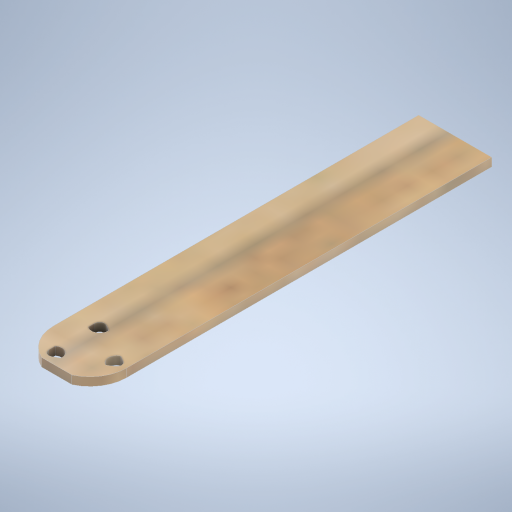
# Autodesk Inventor part: dish_upper
Saved by Autodesk Inventor 2024.1 (Build 281209000, 209)
## iProperties
Created: 2025-09-27
Part Number: dish_upper
Material: 木材 (カエデ材)
Document SubType Name: Modeling
Designer: hibik
Density: 0.67 g/cm^3
Appearance: ナチュラル カエデ材 - 光沢 濃い着色
Author: hibik
Autodesk Inventor part; units mm, degrees
ref_plane "YZ Plane" through (0, 0, 0) normal (1, 0, 0) x (0, 1, 0)
ref_plane "XZ Plane" through (0, 0, 0) normal (0, 1, 0) x (-1, 0, 0)
ref_plane "XY Plane" through (0, 0, 0) normal (0, 0, 1) x (1, 0, 0)
sketch "スケッチ1" plane through (0, 0, 0) normal (0, 1, 0) x (-1, 0, 0)
  circle A0 centre (0, 0) radius 11
  line L0 (11, 10) -> (-11, 10)
  line L1 (-11, 10) -> (-11, -10)
  line L2 (-11, -10) -> (11, -10)
  line L3 (11, -10) -> (11, 10)
  line L4 (11, -10) -> (-11, -10)
  line L5 (-11, -10) -> (-11, -110)
  line L6 (-11, -110) -> (11, -110)
  line L7 (11, -110) -> (11, -10)
  circle A1 centre (0, 0) radius 8 construction
  circle A2 centre (-8, 0) radius 1.5
  circle A3 centre (4, -6.9282) radius 1.5
  circle A4 centre (4, 6.9282) radius 1.5
  line L8 (3.25, 8.2272) -> (-8.75, 1.299)
  line L9 (-8.75, -1.299) -> (3.25, -8.2272)
  line L10 (5.5, -6.9282) -> (5.5, 6.9282)
  circle A5 centre (4, -6.9282) radius 2.5
  circle A6 centre (4, 6.9282) radius 2.5
  circle A7 centre (-8, 0) radius 2.5
  point P0 (11, 0)
  point P1 (11, 0)
  point P2 (4.5826, 10)
  point P3 (-4.5826, 10)
  point P4 (-11, 0)
  point P5 (-7.0179, 2.299)
  point P6 (-7.0179, -2.299)
  point P7 (1.5179, -7.2272)
  point P8 (5.5, -4.9282)
  point P9 (5.5, 4.9282)
  point P10 (1.5179, 7.2272)
  dimension "d3" = 16
  dimension "d0" = 22
  dimension "d1" = 20
  dimension "d2" = 100
  dimension "d4" = 3
  dimension "d7" = 360
  dimension "d11" = 5
  constraints: 22 end point, 7 centre point, 7 tangent, 6 point on circle, 5 coincident, 4 parallel, 3 horizontal alignment, 2 equal radius, 2 horizontal, 2 perpendicular, 1 collinear, 1 midpoint, 1 vertical, 9 other
  measures "d0" diameter of A0
  measures "d1" distance of L2.end L0.start
  measures "d2" distance of L5.end L4.end
  measures "d4" diameter of A2
  measures "d11" diameter of A5
extrude "押し出し1" add sketch "スケッチ1" along normal blind 2.5 contours A0 L2 L0 | L3 L2 A0 | L2 L7 L6 L5 A0 | A0 L2 | L2 L1 A0 | A2 L9 A7 L8 | L8 A6 L10 A5 L9 A7 | A6 L10 A4 L8 | L9 A3 L10 A5 picked at (-7.7924, -2.0224) picked at (2.1405, 7.7484) picked at (2.1405, -7.7484)
